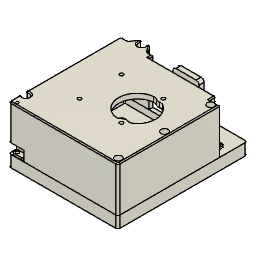
Rover Print (Autodesk Fusion 360 design; units mm, degrees)
Autodesk Fusion 360 part; units mm, degrees
sketch "Sketch1" plane through (0, 0, 0) normal (0, 1, 0) x (1, 0, 0)
  circle A0 centre (-11.34, -55.5844) radius 2
  circle A1 centre (48.2127, -47.8014) radius 2
  circle A2 centre (22.7534, 34.9922) radius 2
  circle A3 centre (-33.3857, 4.4929) radius 2
  line L0 (-55, 25) -> (10, 25)
  line L1 (10, 25) -> (18.6466, 42.3538)
  line L2 (18.6466, 42.3538) -> (53.4157, 42.3538)
  line L3 (53.4157, 42.3538) -> (53.4157, -86.2434)
  line L4 (53.4157, -86.2434) -> (-55, -86.2434)
  line L5 (-55, -86.2434) -> (-55, 25)
  circle A4 centre (48.2127, -47.8014) radius 3.5
  circle A5 centre (-11.34, -55.5844) radius 3.5
  circle A6 centre (-33.3857, 4.4929) radius 3.5
  circle A7 centre (22.7534, 34.9922) radius 3.5
  line L6 (-48, 25) -> (-43, 32)
  line L7 (-43, 32) -> (-33, 32)
  line L8 (-33, 32) -> (-28, 25)
  dimension "d1" = 4
  dimension "d2" = 4
  dimension "d3" = 4
  dimension "d4" = 4
  dimension "d8" = 7
  dimension "d9" = 7
  dimension "d10" = 7
  dimension "d11" = 7
  dimension "d61" = 7
  dimension "d62" = 5
  dimension "d63" = 5
  dimension "d64" = 20
  constraint horizontal L0
  constraint parallel L0 L2
  constraint perpendicular L2 L3
  constraint perpendicular L3 L4
  constraint perpendicular L0 L5
  constraint concentric A1 A4
  constraint concentric A0 A5
  constraint concentric A3 A6
  constraint concentric A2 A7
  constraint coincident L0 L6.start
  constraint parallel L0 L7
  constraint coincident L0 L8.end
  measures "d1" diameter of A0
  measures "d2" diameter of A1
  measures "d3" diameter of A2
  measures "d4" diameter of A3
  measures "d8" diameter of A4
  measures "d9" diameter of A5
  measures "d10" diameter of A6
  measures "d11" diameter of A7
  measures "d61" distance of L0.start L6.start
  measures "d62" horizontal distance of L6.start L6.end
  measures "d63" horizontal distance of L7.end L8.end
  measures "d64" distance of L6.start L8.end
extrude "Extrude2" add sketch "Sketch1" along normal blind 5 contours L0 L1 L2 L3 L4 L5 | L0 L6 L7 L8 | A4 | A5 | A6 | A7 makes body 1
extrude "Extrude3" add sketch "Sketch1" along normal blind 2 contours A4 | A5 | A6 | A7 bodies 1
sketch "Sketch2" plane through (0, 5, 0) normal (0, 1, 0) x (-1, 0, 0)
  circle A0 centre (-22.7534, -34.9922) radius 2
  circle A1 centre (33.3857, -4.4929) radius 2
  circle A2 centre (11.34, 55.5844) radius 2
  circle A3 centre (-48.2127, 47.8014) radius 2
  line L0 (55, 86.2434) -> (-53.4157, 86.2434)
  line L1 (-53.4157, 86.2434) -> (-53.4157, -42.3538)
  line L2 (-53.4157, -42.3538) -> (-18.6466, -42.3538)
  line L3 (-18.6466, -42.3538) -> (-10, -25)
  line L4 (48, -25) -> (55, -25)
  line L5 (55, -25) -> (55, 86.2434)
  line L6 (47, -21.0566) -> (-43.6, -21.0566)
  line L7 (-43.6, -21.0566) -> (-43.6, 82.2434)
  line L8 (-43.6, 82.2434) -> (47, 82.2434)
  line L9 (47, 82.2434) -> (47, -21.0566)
  line L10 (55, 86.2434) -> (55, -25)
  circle A4 centre (46, -20.0566) radius 1
  circle A5 centre (-42.6, -20.0566) radius 1
  circle A6 centre (-42.6, 81.2434) radius 1
  circle A7 centre (46, 81.2434) radius 1
  line L11 (33, -32) -> (43, -32)
  line L12 (43, -32) -> (48, -25)
  line L13 (-10, -25) -> (28, -25)
  line L14 (28, -25) -> (33, -32)
  line L15 (38, -32) -> (38, -29) construction
  circle A8 centre (38, -29) radius 1.3
  line L16 (-43.6, -21.0566) -> (-43.6, -11.0566) construction
  line L17 (-43.6, -11.0566) -> (-48.6, -11.0566) construction
  circle A9 centre (-48.6, -11.0566) radius 1.3
  line L18 (-48.6, -11.0566) -> (-48.6, 11.9434) construction
  circle A10 centre (-48.6, 11.9434) radius 1.3
  line L19 (-48.6, 11.9434) -> (-48.6, 34.9434) construction
  circle A11 centre (-48.6, 34.9434) radius 1.3
  line L20 (-48.6, 34.9434) -> (-48.6, 57.9434) construction
  circle A12 centre (-48.6, 57.9434) radius 1.3
  line L21 (-48.6, 57.9434) -> (-48.6, 80.9434) construction
  circle A13 centre (-48.6, 80.9434) radius 1.3
  line L22 (47, 82.2434) -> (52, 82.2434) construction
  line L23 (52, 82.2434) -> (52, 72.2434) construction
  circle A14 centre (52, 72.2434) radius 1.3
  dimension "d16" = 90.6
  dimension "d17" = 103.3
  dimension "d18" = 8
  dimension "d19" = 4
  dimension "d20" = 2
  dimension "d65" = 3
  dimension "d66" = 2.6
  dimension "d70" = 10
  dimension "d71" = 5
  dimension "d72" = 2.6
  dimension "d73" = 23
  dimension "d74" = 2.6
  dimension "d75" = 23
  dimension "d76" = 2.6
  dimension "d77" = 23
  dimension "d78" = 2.6
  dimension "d79" = 23
  dimension "d80" = 2.6
  dimension "d81" = 5
  dimension "d82" = 10
  dimension "d83" = 2.6
  constraint horizontal L6
  constraint vertical L7
  constraint horizontal L8
  constraint vertical L9
  constraint tangent L9 A4
  constraint tangent L6 A4
  constraint equal A4 A7
  constraint equal A6 A7
  constraint equal A5 A6
  constraint tangent L6 A5
  constraint tangent L7 A5
  constraint tangent L7 A6
  constraint tangent L8 A6
  constraint tangent L9 A7
  constraint tangent L8 A7
  constraint midpoint L11 L15.start
  constraint perpendicular L11 L15
  constraint coincident L15.end A8.centre
  constraint perpendicular L6 L16
  constraint perpendicular L16 L17
  constraint coincident L17.end A9.centre
  constraint perpendicular L17 L18
  constraint coincident L18.end A10.centre
  constraint parallel L18 L19
  constraint coincident L19.end A11.centre
  constraint parallel L19 L20
  constraint coincident L20.end A12.centre
  constraint parallel L20 L21
  constraint coincident L21.end A13.centre
  constraint perpendicular L9 L22
  constraint perpendicular L22 L23
  constraint coincident L23.end A14.centre
  measures "d16" distance of L6.start L6.end
  measures "d17" distance of L6.start L8.end
  measures "d18" distance of L9 L10
  measures "d19" distance of L0 L8
  measures "d20" diameter of A4
  measures "d65" distance of L15.start L15.end
  measures "d66" diameter of A8
  measures "d70" distance of L6.end L16.end
  measures "d71" distance of L16.end L17.end
  measures "d72" diameter of A9
  measures "d73" distance of L17.end L18.end
  measures "d74" diameter of A10
  measures "d75" distance of L18.end L19.end
  measures "d76" diameter of A11
  measures "d77" distance of L19.end L20.end
  measures "d78" diameter of A12
  measures "d79" distance of L20.end L21.end
  measures "d80" diameter of A13
  measures "d81" distance of L8.end L22.end
  measures "d82" distance of L22.end L23.end
  measures "d83" diameter of A14
extrude "Extrude4" add sketch "Sketch2" along normal blind 6.5 contours L0 L1 L2 L3 L4 L5 L10 L11 L12 L13 L14 | L6 L9 A4 | L6 L7 A5 | L8 L9 A7 | L7 L8 A6 | A8 | A9 | A10 | A11 | A12 | A13 | A14 bodies 1
extrude "Extrude5" cut sketch "Sketch1" against normal blind 9.5 from surface at 11.5 contours A4 | A7 bodies 1
extrude "Extrude6" cut sketch "Sketch1" against normal blind 3 from surface at 5 contours A5 | A6 bodies 1
fillet "Fillet1" radius 2 7 edges at (-55, 8.25, -25) (-55, 2.5, -25) (-55, 5.75, 86.2434) (53.4157, 5.75, 86.2434) (53.4157, 5.75, -42.3538) (18.6466, 5.75, -42.3538) (10, 2.5, -25) on bodies 1
sketch "Sketch3" plane through (0, 11.5, 0) normal (0, 1, 0) x (-1, 0, 0)
  arc A0 (-19.8846, -42.3538) -> (-18.0945, -41.2457) centre (-19.8846, -40.3538) ccw
  line L0 (-18.0945, -41.2457) -> (-10.5521, -26.1081)
  line L1 (48, -25) -> (53, -25)
  arc A1 (53, -25) -> (55, -23) centre (53, -23) ccw
  line L2 (55, -23) -> (55, 84.2434)
  arc A2 (55, 84.2434) -> (53, 86.2434) centre (53, 84.2434) ccw
  line L3 (53, 86.2434) -> (-51.4157, 86.2434)
  arc A3 (-51.4157, 86.2434) -> (-53.4157, 84.2434) centre (-51.4157, 84.2434) ccw
  line L4 (-53.4157, 84.2434) -> (-53.4157, -40.3538)
  arc A4 (-53.4157, -40.3538) -> (-51.4157, -42.3538) centre (-51.4157, -40.3538) ccw
  line L5 (-51.4157, -42.3538) -> (-19.8846, -42.3538)
  arc A5 (46, -21.0566) -> (47, -20.0566) centre (46, -20.0566) ccw
  line L6 (46, -21.0566) -> (-42.6, -21.0566)
  arc A6 (-43.6, -20.0566) -> (-42.6, -21.0566) centre (-42.6, -20.0566) ccw
  line L7 (-43.6, -20.0566) -> (-43.6, 81.2434)
  arc A7 (-42.6, 82.2434) -> (-43.6, 81.2434) centre (-42.6, 81.2434) ccw
  line L8 (-42.6, 82.2434) -> (46, 82.2434)
  arc A8 (47, 81.2434) -> (46, 82.2434) centre (46, 81.2434) ccw
  line L9 (47, 81.2434) -> (47, -20.0566)
  circle A9 centre (-22.7534, -34.9922) radius 3.5
  circle A10 centre (-48.2127, 47.8014) radius 3.5
  line L10 (46, 82.2434) -> (46, 80.7434) construction
  line L11 (46, 80.7434) -> (42, 80.7434) construction
  line L12 (42, 80.7434) -> (52, 80.7434)
  line L13 (52, 80.7434) -> (52, 85.7434)
  line L14 (52, 85.7434) -> (42, 85.7434)
  line L15 (42, 85.7434) -> (42, 80.7434)
  circle A11 centre (49.5, 83.2434) radius 1.6
  circle A12 centre (49.5, 83.2434) radius 1.3
  line L16 (-43.6, -20.0566) -> (-41.6, -20.0566) construction
  line L17 (-41.6, -20.0566) -> (-41.6, -16.0566) construction
  line L18 (-41.6, -16.0566) -> (-46.6, -16.0566)
  line L19 (-46.6, -16.0566) -> (-46.6, -26.0566)
  line L20 (-46.6, -26.0566) -> (-41.6, -26.0566)
  line L21 (-41.6, -26.0566) -> (-41.6, -16.0566)
  circle A13 centre (-44.1, -23.5566) radius 1.6
  circle A14 centre (-44.1, -23.5566) radius 1.3
  arc A15 (-8.762, -25) -> (-10.5521, -26.1081) centre (-8.762, -27) ccw
  line L22 (-8.762, -25) -> (28, -25)
  line L23 (28, -25) -> (33, -32)
  line L24 (33, -32) -> (43, -32)
  line L25 (43, -32) -> (48, -25)
  dimension "d31" = 1.5
  dimension "d32" = 10
  dimension "d33" = 5
  dimension "d34" = 3.2
  dimension "d35" = 2.6
  dimension "d42" = 2
  dimension "d43" = 4
  dimension "d44" = 5
  dimension "d45" = 10
  dimension "d46" = 3.2
  dimension "d47" = 2.6
  dimension "d48" = 2.5
  dimension "d49" = 2.5
  dimension "d50" = 2.5
  dimension "d51" = 2.5
  constraint coincident L8.end A8.end
  constraint perpendicular L8 L10
  constraint perpendicular L10 L11
  constraint horizontal L12
  constraint vertical L13
  constraint horizontal L14
  constraint vertical L15
  constraint concentric A11 A12
  constraint coincident A6.start L7.start
  constraint perpendicular L7 L16
  constraint perpendicular L16 L17
  constraint horizontal L18
  constraint vertical L19
  constraint horizontal L20
  constraint vertical L21
  constraint concentric A13 A14
  measures "d31" distance of L8.end L10.end
  measures "d32" distance of L11.end L12.end
  measures "d33" distance of L11.end L14.end
  measures "d34" diameter of A11
  measures "d35" diameter of A12
  measures "d42" distance of A6.start L16.end
  measures "d43" distance of L16.end L17.end
  measures "d44" distance of L17.end L18.end
  measures "d45" distance of L17.end L20.end
  measures "d46" diameter of A13
  measures "d47" diameter of A14
  measures "d48" distance of L13 A11.centre
  measures "d49" distance of L14 A11.centre
  measures "d50" distance of L20 A13.centre
  measures "d51" distance of L19 A13.centre
extrude "Extrude7" cut sketch "Sketch3" against normal blind 7 contours A12 bodies 1
extrude "Extrude8" add sketch "Sketch3" along normal blind 2 separate body contours L8 A8 L9 L12 L15 | L8 A8 L9 L12 L13 L14 L15 makes body 2
fillet "Fillet2" radius 1 4 edges at (-42, 12.5, 85.7434) (-52, 12.5, 85.7434) (-52, 12.5, 80.7434) (-42, 12.5, 80.7434) on bodies 2
extrude "Extrude9" cut sketch "Sketch3" against normal blind 7 contours A14 bodies 1
extrude "Extrude10" add sketch "Sketch3" along normal blind 2 separate body contours L6 A6 L7 L18 L19 L20 L21 | L6 A6 L7 L18 L21 makes body 3
fillet "Fillet3" radius 1 4 edges at (46.6, 12.5, -16.0566) (41.6, 12.5, -16.0566) (41.6, 12.5, -26.0566) (46.6, 12.5, -26.0566) on bodies 3
fillet "Fillet4" radius 2 6 edges at (-48, 2.5, -25) (-48, 8.25, -25) (-43, 5.75, -32) (-33, 5.75, -32) (-28, 2.5, -25) (-28, 8.25, -25) on bodies 1
extrude "Extrude11" cut sketch "Sketch2" against normal blind 7 from surface at 6.5 contours A8 bodies 1
extrude "Extrude12" cut sketch "Sketch2" against normal blind 7 from surface at 6.5 contours A9 | A10 | A11 | A12 | A13 | A14 bodies 1
sketch "Sketch4" plane through (0, 11.5, 0) normal (0, 1, 0) x (-1, 0, 0)
  circle A0 centre (-48.6, 34.9434) radius 1.3
  circle A1 centre (52, 72.2434) radius 1.3
  circle A2 centre (-48.6, 11.9434) radius 1.3
  circle A3 centre (-48.6, 57.9434) radius 1.3
  circle A4 centre (-48.6, 80.9434) radius 1.3
  circle A5 centre (-48.6, -11.0566) radius 1.3
  circle A6 centre (38, -29) radius 1.3
  circle A7 centre (-44.1, -23.5566) radius 1.3
  circle A8 centre (49.5, 83.2434) radius 1.3
  arc A9 (32.4018, -31.1625) -> (34.0292, -32) centre (34.0292, -30) ccw
  line L0 (34.0292, -32) -> (41.9708, -32)
  arc A10 (41.9708, -32) -> (43.5982, -31.1625) centre (41.9708, -30) ccw
  line L1 (43.5982, -31.1625) -> (47.4018, -25.8375)
  arc A11 (49.0292, -25) -> (47.4018, -25.8375) centre (49.0292, -27) ccw
  line L2 (49.0292, -25) -> (53, -25)
  arc A12 (53, -25) -> (55, -23) centre (53, -23) ccw
  line L3 (55, -23) -> (55, 84.2434)
  arc A13 (55, 84.2434) -> (53, 86.2434) centre (53, 84.2434) ccw
  line L4 (53, 86.2434) -> (-51.4157, 86.2434)
  arc A14 (-51.4157, 86.2434) -> (-53.4157, 84.2434) centre (-51.4157, 84.2434) ccw
  line L5 (-53.4157, 84.2434) -> (-53.4157, -40.3538)
  arc A15 (-53.4157, -40.3538) -> (-51.4157, -42.3538) centre (-51.4157, -40.3538) ccw
  line L6 (-51.4157, -42.3538) -> (-19.8846, -42.3538)
  arc A16 (-19.8846, -42.3538) -> (-18.0945, -41.2457) centre (-19.8846, -40.3538) ccw
  line L7 (-18.0945, -41.2457) -> (-10.5521, -26.1081)
  arc A17 (-8.762, -25) -> (-10.5521, -26.1081) centre (-8.762, -27) ccw
  line L8 (-8.762, -25) -> (26.9708, -25)
  arc A18 (28.5982, -25.8375) -> (26.9708, -25) centre (26.9708, -27) ccw
  line L9 (28.5982, -25.8375) -> (32.4018, -31.1625)
  arc A19 (46, -21.0566) -> (47, -20.0566) centre (46, -20.0566) ccw
  line L10 (46, -21.0566) -> (-42.6, -21.0566)
  arc A20 (-43.6, -20.0566) -> (-42.6, -21.0566) centre (-42.6, -20.0566) ccw
  line L11 (-43.6, -20.0566) -> (-43.6, 81.2434)
  arc A21 (-42.6, 82.2434) -> (-43.6, 81.2434) centre (-42.6, 81.2434) ccw
  line L12 (-42.6, 82.2434) -> (46, 82.2434)
  arc A22 (47, 81.2434) -> (46, 82.2434) centre (46, 81.2434) ccw
  line L13 (47, 81.2434) -> (47, -20.0566)
  circle A23 centre (-22.7534, -34.9922) radius 3.5
  circle A24 centre (-48.2127, 47.8014) radius 3.5
  line L14 (47, -20.0566) -> (55, -20.0566)
  line L15 (23, -21.0566) -> (23, -25)
  line L16 (-43.6, -15.0178) -> (-53.4157, -15.0178)
  line L17 (47, 59.5753) -> (55, 59.5753)
  circle A25 centre (52, 72.2434) radius 3.5
  circle A26 centre (38, -29) radius 3.5
  circle A27 centre (-48.6, -11.0566) radius 3.5
  circle A28 centre (-48.6, 34.9434) radius 3.5
  circle A29 centre (-48.6, 80.9434) radius 3.5
  dimension "d117" = 7
  dimension "d118" = 7
  dimension "d119" = 7
  dimension "d120" = 7
  dimension "d121" = 7
  dimension "d133" = 24
  constraint coincident A19.end L13.end
  constraint coincident L3 L14.end
  constraint perpendicular L3 L14
  constraint coincident L10 L15.start
  constraint coincident L8 L15.end
  constraint perpendicular L8 L15
  constraint coincident L11 L16.start
  constraint coincident L5 L16.end
  constraint perpendicular L5 L16
  constraint coincident L13 L17.start
  constraint coincident L3 L17.end
  constraint perpendicular L3 L17
  constraint concentric A1 A25
  constraint concentric A6 A26
  constraint concentric A5 A27
  constraint concentric A0 A28
  constraint concentric A4 A29
  measures "d117" diameter of A25
  measures "d118" diameter of A26
  measures "d119" diameter of A27
  measures "d120" diameter of A28
  measures "d121" diameter of A29
  measures "d133" horizontal distance of A19.end L15.start
extrude "Extrude13" add sketch "Sketch4" along normal blind 40 separate body contours A2 | A3 | A9 L0 A10 L1 A11 L2 A12 L3 L8 A18 L9 A19 L10 L14 L15 A26 | L0 A26 | L3 A13 L4 A14 L5 L11 A21 L12 A22 L13 L16 L17 A25 | L3 A25 | A24 | A27 | A28 | A29 picked at (37.9676, -31.4321) picked at (54.4333, 72.2434) makes body 4 at (-38.3333, 24.8333, -21.0566) makes body 5 at (-18.1948, 24.8333, 86.2434)
extrude "Extrude14" add sketch "Sketch4" along normal blind 5 from surface at 40 contours A2 | A3 | A9 L0 A10 L1 A11 L2 A12 L3 L8 A18 L9 A19 L10 L14 L15 A26 | L0 A26 | A19 L10 A20 L11 A21 L12 A22 L13 | L3 L13 L14 L17 | L3 A13 L4 A14 L5 L11 A21 L12 A22 L13 L16 L17 A25 | L3 A25 | A24 | A27 | A28 | A29 picked at (37.9676, -31.4321) picked at (54.4333, 72.2434) bodies 4 5
sketch "Sketch5" plane through (0, 51.5, 0) normal (0, -1, 0) x (1, 0, 0)
  line L0 (-55, -20.0566) -> (-47, -20.0566)
  arc A0 (-47, -20.0566) -> (-46, -21.0566) centre (-46, -20.0566) ccw
  line L1 (-46, -21.0566) -> (-23, -21.0566)
  line L2 (-23, -21.0566) -> (42.6, -21.0566)
  arc A1 (42.6, -21.0566) -> (43.6, -20.0566) centre (42.6, -20.0566) ccw
  line L3 (43.6, -20.0566) -> (43.6, -15.0178)
  line L4 (43.6, -15.0178) -> (43.6, 81.2434)
  arc A2 (43.6, 81.2434) -> (42.6, 82.2434) centre (42.6, 81.2434) ccw
  line L5 (42.6, 82.2434) -> (-46, 82.2434)
  arc A3 (-46, 82.2434) -> (-47, 81.2434) centre (-46, 81.2434) ccw
  line L6 (-47, 81.2434) -> (-47, 59.5753)
  line L7 (-47, 59.5753) -> (-55, 59.5753)
  line L8 (-55, 59.5753) -> (-55, -20.0566)
  line L9 (-1.1187, -54.3751) -> (-1.1187, 110.6249) construction
  circle A4 centre (-1.1187, 28.1249) radius 29.5 construction
  line L10 (-1.1187, 28.1249) -> (19.7409, 7.2652) construction
  line L11 (-1.1187, 28.1249) -> (20, 28.1249) construction
  circle A5 centre (19.7409, 7.2652) radius 1.75
  circle A6 centre (19.7409, 48.9845) radius 1.75
  circle A7 centre (-21.9784, 48.9845) radius 1.75
  circle A8 centre (-21.9784, 7.2652) radius 1.75
  dimension "d92" = 59
  dimension "d93" = 45
  dimension "d94" = 3.5
  dimension "d96" = 360
  constraint perpendicular L5 L9
  constraint midpoint L9 A4.centre
  constraint horizontal L11
  constraint coincident A4.centre L10.start
  constraint coincident A4 L10.end
  constraint coincident L10.end A5.centre
  measures "d92" diameter of A4
  measures "d93" angle of L10 L11
  measures "d94" diameter of A5
extrude "Extrude15" cut sketch "Sketch5" along normal blind 20 from surface at -5 contours A5 | A6 | A7 | A8 bodies 4
sketch "Sketch6" plane through (0, 56.5, 0) normal (0, 1, 0) x (-1, 0, 0)
  circle A0 centre (21.9784, 7.2652) radius 1.75
  circle A1 centre (21.9784, 48.9845) radius 1.75
  circle A2 centre (-19.7409, 7.2652) radius 1.75
  circle A3 centre (-19.7409, 48.9845) radius 1.75
  circle A4 centre (49.5, 83.2434) radius 1.3
  circle A5 centre (52, 72.2434) radius 1.3
  circle A6 centre (-48.6, 80.9434) radius 1.3
  circle A7 centre (-48.6, -11.0566) radius 1.3
  circle A8 centre (38, -29) radius 1.3
  circle A9 centre (-48.6, 34.9434) radius 1.3
  line L0 (-43.6, -15.0178) -> (-43.6, -20.0566)
  arc A10 (-43.6, -20.0566) -> (-42.6, -21.0566) centre (-42.6, -20.0566) ccw
  line L1 (-42.6, -21.0566) -> (23, -21.0566)
  line L2 (23, -21.0566) -> (23, -25)
  line L3 (23, -25) -> (26.9708, -25)
  arc A11 (28.5982, -25.8375) -> (26.9708, -25) centre (26.9708, -27) ccw
  line L4 (28.5982, -25.8375) -> (32.4018, -31.1625)
  arc A12 (32.4018, -31.1625) -> (34.0292, -32) centre (34.0292, -30) ccw
  line L5 (34.0292, -32) -> (41.9708, -32)
  arc A13 (41.9708, -32) -> (43.5982, -31.1625) centre (41.9708, -30) ccw
  line L6 (43.5982, -31.1625) -> (47.4018, -25.8375)
  arc A14 (49.0292, -25) -> (47.4018, -25.8375) centre (49.0292, -27) ccw
  line L7 (49.0292, -25) -> (53, -25)
  arc A15 (53, -25) -> (55, -23) centre (53, -23) ccw
  line L8 (55, -23) -> (55, 84.2434)
  arc A16 (55, 84.2434) -> (53, 86.2434) centre (53, 84.2434) ccw
  line L9 (53, 86.2434) -> (-51.4157, 86.2434)
  arc A17 (-51.4157, 86.2434) -> (-53.4157, 84.2434) centre (-51.4157, 84.2434) ccw
  line L10 (-53.4157, 84.2434) -> (-53.4157, -15.0178)
  line L11 (-53.4157, -15.0178) -> (-43.6, -15.0178)
  circle A18 centre (-48.6, -11.0566) radius 3.5
  circle A19 centre (-48.6, 11.9434) radius 3.5
  circle A20 centre (-48.6, 34.9434) radius 3.5
  circle A21 centre (-48.6, 57.9434) radius 3.5
  circle A22 centre (-48.6, 80.9434) radius 3.5
  circle A23 centre (52, 72.2434) radius 3.5
  circle A24 centre (38, -29) radius 3.5
  dimension "d100" = 7
  dimension "d101" = 7
  dimension "d102" = 7
  dimension "d103" = 7
  dimension "d104" = 7
  dimension "d105" = 7
  dimension "d108" = 7
  constraint concentric A7 A18
  constraint concentric A9 A20
  constraint concentric A6 A22
  constraint concentric A5 A23
  constraint concentric A8 A24
  measures "d100" diameter of A18
  measures "d101" diameter of A19
  measures "d102" diameter of A20
  measures "d103" diameter of A21
  measures "d104" diameter of A22
  measures "d105" diameter of A23
  measures "d108" diameter of A24
sketch "Sketch7" plane through (0, 11.5, 0) normal (0, -1, 0) x (1, 0, 0)
  circle A0 centre (-52, 72.2434) radius 1.3
  circle A1 centre (48.6, -11.0566) radius 1.3
  circle A2 centre (48.6, 80.9434) radius 1.3
  circle A3 centre (48.6, 34.9434) radius 1.3
  circle A4 centre (-49.5, 83.2434) radius 1.3
  line L0 (-47, 59.5753) -> (-47, 81.2434)
  arc A5 (-46, 82.2434) -> (-47, 81.2434) centre (-46, 81.2434) ccw
  line L1 (-46, 82.2434) -> (42.6, 82.2434)
  arc A6 (43.6, 81.2434) -> (42.6, 82.2434) centre (42.6, 81.2434) ccw
  line L2 (43.6, 81.2434) -> (43.6, -15.0178)
  line L3 (43.6, -15.0178) -> (53.4157, -15.0178)
  line L4 (53.4157, -15.0178) -> (53.4157, 84.2434)
  arc A7 (53.4157, 84.2434) -> (51.4157, 86.2434) centre (51.4157, 84.2434) ccw
  line L5 (51.4157, 86.2434) -> (-53, 86.2434)
  arc A8 (-53, 86.2434) -> (-55, 84.2434) centre (-53, 84.2434) ccw
  line L6 (-55, 84.2434) -> (-55, 59.5753)
  line L7 (-55, 59.5753) -> (-47, 59.5753)
  line L8 (-47, 79) -> (-55, 79)
  line L9 (-40.1248, 82.2434) -> (-40.1248, 86.2434)
  constraint coincident L0 L8.start
  constraint coincident L6 L8.end
  constraint perpendicular L6 L8
  constraint coincident L1 L9.start
  constraint coincident L5 L9.end
  constraint perpendicular L5 L9
extrude "Extrude16" cut sketch "Sketch7" against normal blind 10 contours A4 | L0 A5 L1 L5 A8 L6 L8 L9 bodies 4
extrude "Extrude17" cut sketch "Sketch6" against normal blind 45 contours L8 A23 | L5 A24 | A18 | A20 | A22 picked at (54.4333, 72.2434) picked at (37.9676, -31.4321) bodies 4
extrude "Extrude18" add sketch "Sketch4" along normal blind 2 contours L0 A26 | L3 A25 | A27 | A28 | A29 picked at (37.9676, -31.4321) picked at (54.4333, 72.2434) bodies 4
fillet "Fillet5" radius 1 2 edges at (-55, 34, 70.4406) (-55, 34, 74.0462) on bodies 4
fillet "Fillet6" radius 1 2 edges at (-36.1972, 34, -32) (-39.8028, 34, -32) on bodies 4
fillet "Fillet7" radius 1 26 edges at (-23, 56.5, -23.0283) (43.6, 56.5, -17.5372) (43.3071, 56.5, -20.7637) (9.8, 56.5, -21.0566) (-24.9854, 56.5, -25) (-27.8859, 56.5, -25.2217) (-30.5, 56.5, -28.5) (-33.06, 56.5, -31.7494) (-34.8011, 56.5, -31.5512) (-38, 56.5, -25.5) (-41.1989, 56.5, -31.5512) (-42.94, 56.5, -31.7494) (-45.5, 56.5, -28.5) (-48.1141, 56.5, -25.2217) (-51.0146, 56.5, -25) (-54.4142, 56.5, -24.4142) (-55, 56.5, 22.6061) (-54.527, 56.5, 69.0621) (-48.5, 56.5, 72.2434) (-54.527, 56.5, 75.4247) (-55, 56.5, 80.259) (-54.4142, 56.5, 85.6576) (-0.7922, 56.5, 86.2434) (52.8299, 56.5, 85.6576) (53.4157, 56.5, 34.6128) (48.5078, 56.5, -15.0178) on bodies 4
sketch "Sketch8" plane through (0, 56.5, 0) normal (0, 1, 0) x (-1, 0, 0)
  line L0 (-52.4157, -14.0178) -> (-50.4658, -14.0178)
  arc A0 (-46.7342, -14.0178) -> (-50.4658, -14.0178) centre (-48.6, -11.0566) ccw
  line L1 (-46.7342, -14.0178) -> (-42.6, -14.0178)
  line L2 (-42.6, -14.0178) -> (-42.6, -20.0566)
  line L3 (-42.6, -20.0566) -> (24, -20.0566)
  line L4 (24, -20.0566) -> (24, -24)
  line L5 (24, -24) -> (26.9708, -24)
  arc A1 (29.412, -25.2563) -> (26.9708, -24) centre (26.9708, -27) ccw
  line L6 (29.412, -25.2563) -> (33.2155, -30.5812)
  arc A2 (33.2155, -30.5812) -> (33.9679, -30.9981) centre (34.0292, -30) ccw
  arc A3 (42.0321, -30.9981) -> (33.9679, -30.9981) centre (38, -29) ccw
  arc A4 (42.0321, -30.9981) -> (42.7845, -30.5812) centre (41.9708, -30) ccw
  line L7 (42.7845, -30.5812) -> (46.588, -25.2563)
  arc A5 (49.0292, -24) -> (46.588, -25.2563) centre (49.0292, -27) ccw
  line L8 (49.0292, -24) -> (53, -24)
  arc A6 (53, -24) -> (54, -23) centre (53, -23) ccw
  line L9 (54, -23) -> (54, 68.2123)
  arc A7 (54, 76.2746) -> (54, 68.2123) centre (52, 72.2434) ccw
  line L10 (54, 76.2746) -> (54, 84.2434)
  arc A8 (54, 84.2434) -> (53, 85.2434) centre (53, 84.2434) ccw
  line L11 (53, 85.2434) -> (-51.4157, 85.2434)
  arc A9 (-51.4157, 85.2434) -> (-52.4157, 84.2434) centre (-51.4157, 84.2434) ccw
  line L12 (-52.4157, 84.2434) -> (-52.4157, -14.0178)
  circle A10 centre (-48.6, 34.9434) radius 3.5
  circle A11 centre (-48.6, 80.9434) radius 3.5
  circle A12 centre (21.9784, 7.2652) radius 1.75
  circle A13 centre (21.9784, 48.9845) radius 1.75
  circle A14 centre (-19.7409, 7.2652) radius 1.75
  circle A15 centre (-19.7409, 48.9845) radius 1.75
  circle A16 centre (49.5, 83.2434) radius 1.3
  line L13 (-43.6, 82.2) -> (-33.6, 82.2) construction
  line L14 (-33.6, 82.2) -> (-33.6, 47.2) construction
  line L15 (-33.6, 47.2) -> (3.4, 47.2) construction
  line L16 (3.4, 47.2) -> (3.4, 10.2) construction
  line L17 (3.4, 10.2) -> (-33.6, 10.2) construction
  line L18 (-33.6, 10.2) -> (-33.6, 47.2) construction
  circle A17 centre (-15.1, 28.7) radius 18.5
  circle A18 centre (-19.7409, 48.9845) radius 5
  circle A19 centre (-19.7409, 7.2652) radius 5
  dimension "d124" = 10
  dimension "d125" = 35
  dimension "d126" = 37
  dimension "d127" = 37
  dimension "d128" = 37
  dimension "d173" = 10
  dimension "d174" = 10
  constraint parallel L11 L13
  constraint perpendicular L13 L14
  constraint horizontal L15
  constraint vertical L16
  constraint horizontal L17
  constraint vertical L18
  constraint concentric A15 A18
  constraint concentric A14 A19
  measures "d124" distance of L13.start L13.end
  measures "d125" distance of L13.end L14.end
  measures "d126" distance of L14.end L15.end
  measures "d127" distance of L14.end L17.end
  measures "d128" diameter of A17
  measures "d173" diameter of A18
  measures "d174" diameter of A19
extrude "Extrude19" cut sketch "Sketch8" against normal blind 10 contours A17 A18 A19 bodies 4
fillet "Fillet8" radius 5 3 edges at (23.171, 54, 45.3466) (23.171, 54, 45.3466) (15.0703, 54, 47.2) on bodies 4
sketch "Sketch9" plane through (0, 11.5, 0) normal (0, 1, 0) x (-1, 0, 0)
  circle A0 centre (-48.6, 34.9434) radius 1.3
  circle A1 centre (52, 72.2434) radius 1.3
  circle A2 centre (-48.6, 11.9434) radius 1.3
  circle A3 centre (-48.6, 57.9434) radius 1.3
  circle A4 centre (-48.6, 80.9434) radius 1.3
  circle A5 centre (-48.6, -11.0566) radius 1.3
  circle A6 centre (38, -29) radius 1.3
  circle A7 centre (-44.1, -23.5566) radius 1.3
  circle A8 centre (49.5, 83.2434) radius 1.3
  arc A9 (32.4018, -31.1625) -> (34.0292, -32) centre (34.0292, -30) ccw
  line L0 (34.0292, -32) -> (41.9708, -32)
  arc A10 (41.9708, -32) -> (43.5982, -31.1625) centre (41.9708, -30) ccw
  line L1 (43.5982, -31.1625) -> (47.4018, -25.8375)
  arc A11 (49.0292, -25) -> (47.4018, -25.8375) centre (49.0292, -27) ccw
  line L2 (49.0292, -25) -> (53, -25)
  arc A12 (53, -25) -> (55, -23) centre (53, -23) ccw
  line L3 (55, -23) -> (55, 84.2434)
  arc A13 (55, 84.2434) -> (53, 86.2434) centre (53, 84.2434) ccw
  line L4 (53, 86.2434) -> (-51.4157, 86.2434)
  arc A14 (-51.4157, 86.2434) -> (-53.4157, 84.2434) centre (-51.4157, 84.2434) ccw
  line L5 (-53.4157, 84.2434) -> (-53.4157, -40.3538)
  arc A15 (-53.4157, -40.3538) -> (-51.4157, -42.3538) centre (-51.4157, -40.3538) ccw
  line L6 (-51.4157, -42.3538) -> (-19.8846, -42.3538)
  arc A16 (-19.8846, -42.3538) -> (-18.0945, -41.2457) centre (-19.8846, -40.3538) ccw
  line L7 (-18.0945, -41.2457) -> (-10.5521, -26.1081)
  arc A17 (-8.762, -25) -> (-10.5521, -26.1081) centre (-8.762, -27) ccw
  line L8 (-8.762, -25) -> (26.9708, -25)
  arc A18 (28.5982, -25.8375) -> (26.9708, -25) centre (26.9708, -27) ccw
  line L9 (28.5982, -25.8375) -> (32.4018, -31.1625)
  arc A19 (46, -21.0566) -> (47, -20.0566) centre (46, -20.0566) ccw
  line L10 (46, -21.0566) -> (-42.6, -21.0566)
  arc A20 (-43.6, -20.0566) -> (-42.6, -21.0566) centre (-42.6, -20.0566) ccw
  line L11 (-43.6, -20.0566) -> (-43.6, 81.2434)
  arc A21 (-42.6, 82.2434) -> (-43.6, 81.2434) centre (-42.6, 81.2434) ccw
  line L12 (-42.6, 82.2434) -> (46, 82.2434)
  arc A22 (47, 81.2434) -> (46, 82.2434) centre (46, 81.2434) ccw
  line L13 (47, 81.2434) -> (47, -20.0566)
  circle A23 centre (-22.7534, -34.9922) radius 3.5
  circle A24 centre (-48.2127, 47.8014) radius 3.5
  line L14 (0, 0) -> (0, -36) construction
  constraint coincident L14.start origin
  constraint vertical L14
sketch "Sketch10" plane through (0, 0, -25) normal (0, 0, -1) x (-1, 0, 0)
  line L0 (26.9708, 5) -> (26.9708, 11.5)
  line L1 (26.9708, 11.5) -> (-8.762, 11.5)
  line L2 (-8.762, 11.5) -> (-8.762, 5)
  line L3 (-8.762, 5) -> (26.9708, 5)
  circle A0 centre (-4, 8) radius 1.3
  line L4 (-4, 8) -> (16, 8) construction
  circle A1 centre (16, 8) radius 1.3
  line L5 (6, 8) -> (6, 3) construction
  circle A2 centre (6, 3) radius 1.3
  line L6 (6, 0) -> (0, 0)
  line L7 (0, 0) -> (-7, 5)
  line L8 (12, 0) -> (19, 5)
  line L9 (6, 0) -> (12, 0)
  line L10 (-7, 5) -> (-7, 11.5)
  line L11 (19, 5) -> (19, 11.5)
  dimension "d134" = 2.6
  dimension "d135" = 20
  dimension "d136" = 2.6
  dimension "d137" = 5
  dimension "d138" = 2.6
  constraint coincident A0.centre L4.start
  constraint horizontal L4
  constraint coincident L4.end A1.centre
  constraint midpoint L4 L5.start
  constraint perpendicular L4 L5
  constraint coincident L5.end A2.centre
  constraint coincident L6.end L7.start
  constraint horizontal L6
  constraint coincident L3 L7.end
  constraint symmetric L5 L6.start L9.start
  constraint symmetric L5 L6.end L8.start
  constraint symmetric L5 L7.end L8.end
  constraint coincident L1 L10.end
  constraint perpendicular L1 L10
  constraint coincident L1 L11.end
  constraint perpendicular L1 L11
  measures "d134" diameter of A0
  measures "d135" distance of A0.centre L4.end
  measures "d136" diameter of A1
  measures "d137" distance of L5.start L5.end
  measures "d138" diameter of A2
extrude "Extrude20" add sketch "Sketch10" along normal blind 15 separate body contours L3 L6 L7 L8 L9 | L1 L3 L10 L11 | A0 | A1 | A2 makes body 6
move_body "Move1" bodies 6 to x (1, 0, 0) y (0, 1, 0) z (0, 0, 1) at (6, 0, 0)
combine "Combine1" operation add target body 1 tool bodies 6
sketch "Sketch11" plane through (0, 11.5, 0) normal (0, 1, 0) x (-1, 0, 0)
  circle A0 centre (-48.2127, 47.8014) radius 3.5
  circle A1 centre (-22.7534, -34.9922) radius 3.5
  arc A2 (46, -21.0566) -> (47, -20.0566) centre (46, -20.0566) ccw
  line L0 (46, -21.0566) -> (-42.6, -21.0566)
  arc A3 (-43.6, -20.0566) -> (-42.6, -21.0566) centre (-42.6, -20.0566) ccw
  line L1 (-43.6, -20.0566) -> (-43.6, 81.2434)
  arc A4 (-42.6, 82.2434) -> (-43.6, 81.2434) centre (-42.6, 81.2434) ccw
  line L2 (-42.6, 82.2434) -> (46, 82.2434)
  arc A5 (47, 81.2434) -> (46, 82.2434) centre (46, 81.2434) ccw
  line L3 (47, 81.2434) -> (47, -20.0566)
  line L4 (-13, -31.021) -> (-13, -40)
  line L5 (-13, -40) -> (13, -40)
  line L6 (13, -40) -> (13, -25)
  line L7 (13, -25) -> (26.9708, -25)
  arc A6 (28.5982, -25.8375) -> (26.9708, -25) centre (26.9708, -27) ccw
  line L8 (28.5982, -25.8375) -> (32.4018, -31.1625)
  arc A7 (32.4018, -31.1625) -> (34.0292, -32) centre (34.0292, -30) ccw
  line L9 (34.0292, -32) -> (41.9708, -32)
  arc A8 (41.9708, -32) -> (43.5982, -31.1625) centre (41.9708, -30) ccw
  line L10 (43.5982, -31.1625) -> (47.4018, -25.8375)
  arc A9 (49.0292, -25) -> (47.4018, -25.8375) centre (49.0292, -27) ccw
  line L11 (49.0292, -25) -> (53, -25)
  arc A10 (53, -25) -> (55, -23) centre (53, -23) ccw
  line L12 (55, -23) -> (55, 84.2434)
  arc A11 (55, 84.2434) -> (53, 86.2434) centre (53, 84.2434) ccw
  line L13 (53, 86.2434) -> (-51.4157, 86.2434)
  arc A12 (-51.4157, 86.2434) -> (-53.4157, 84.2434) centre (-51.4157, 84.2434) ccw
  line L14 (-53.4157, 84.2434) -> (-53.4157, -40.3538)
  arc A13 (-53.4157, -40.3538) -> (-51.4157, -42.3538) centre (-51.4157, -40.3538) ccw
  line L15 (-51.4157, -42.3538) -> (-19.8846, -42.3538)
  arc A14 (-19.8846, -42.3538) -> (-18.0945, -41.2457) centre (-19.8846, -40.3538) ccw
  line L16 (-18.0945, -41.2457) -> (-13, -31.021)
  circle A15 centre (49.5, 83.2434) radius 1.3
  circle A16 centre (-44.1, -23.5566) radius 1.3
  circle A17 centre (38, -29) radius 1.3
  circle A18 centre (-48.6, -11.0566) radius 1.3
  circle A19 centre (-48.6, 80.9434) radius 1.3
  circle A20 centre (-48.6, 57.9434) radius 1.3
  circle A21 centre (-48.6, 11.9434) radius 1.3
  circle A22 centre (52, 72.2434) radius 1.3
  circle A23 centre (-48.6, 34.9434) radius 1.3
  circle A24 centre (0, -31) radius 1.3
  line L17 (13, -40) -> (13, -35) construction
  line L18 (13, -35) -> (-13, -35)
  line L19 (0, -35) -> (0, -31) construction
  line L20 (0, -31) -> (-9, -31) construction
  circle A25 centre (-9, -31) radius 1.3
  line L21 (0, -31) -> (9, -31) construction
  circle A26 centre (9, -31) radius 1.3
  line L22 (-13, -35) -> (-13, -25)
  line L23 (-13, -25) -> (13, -25)
  dimension "d141" = 2.6
  dimension "d142" = 5
  dimension "d143" = 4
  dimension "d144" = 2.6
  dimension "d145" = 9
  dimension "d146" = 2.6
  dimension "d147" = 10
  constraint coincident L5.end L6.start
  constraint perpendicular L5 L17
  constraint coincident L4 L18.end
  constraint perpendicular L4 L18
  constraint midpoint L18 L19.start
  constraint perpendicular L18 L19
  constraint coincident A24.centre L19.end
  constraint perpendicular L19 L20
  constraint coincident L20.end A25.centre
  constraint perpendicular L19 L21
  constraint coincident L21.end A26.centre
  constraint perpendicular L18 L22
  constraint coincident L6.end L7.start
  measures "d141" diameter of A24
  measures "d142" distance of L5.end L17.end
  measures "d143" distance of L19.start A24.centre
  measures "d144" diameter of A25
  measures "d145" distance of A24.centre L21.end
  measures "d146" diameter of A26
  measures "d147" distance of L18.end L22.end
extrude "Extrude21" add sketch "Sketch11" along normal blind 5 contours L4 L6 L18 L22 L23 | L4 L5 L6 L18 bodies 1
extrude "Extrude22" add sketch "Sketch11" along normal blind 35 contours L4 L5 L6 L18 bodies 1
sketch "Sketch12" plane through (0, 0, -40) normal (0, 0, -1) x (-1, 0, 0)
  line L0 (-13, 46.5) -> (-13, 5)
  line L1 (-13, 5) -> (-6, 0)
  line L2 (-6, 0) -> (6, 0)
  line L3 (6, 0) -> (13, 5)
  line L4 (13, 5) -> (13, 46.5)
  line L5 (13, 46.5) -> (-13, 46.5)
  line L6 (0, 46.5) -> (0, 41.5) construction
  line L7 (0, 41.5) -> (-42.5, 41.5) construction
  line L8 (-42.5, 41.5) -> (42.5, 41.5) construction
  line L9 (42.5, 41.5) -> (42.5, 17.5) construction
  line L10 (42.5, 17.5) -> (-42.5, 17.5) construction
  line L11 (-42.5, 17.5) -> (-42.5, 41.5) construction
  dimension "d152" = 5
  dimension "d153" = 42.5
  dimension "d154" = 85
  dimension "d155" = 24
  constraint midpoint L5 L6.start
  constraint perpendicular L5 L6
  constraint perpendicular L6 L7
  constraint horizontal L8
  constraint vertical L9
  constraint horizontal L10
  constraint vertical L11
  measures "d152" distance of L6.start L6.end
  measures "d153" distance of L6.end L7.end
  measures "d154" distance of L7.end L8.end
  measures "d155" distance of L7.end L10.end
sketch "Sketch13" plane through (0, 0, -40) normal (0, 0, -1) x (-1, 0, 0)
  line L0 (-13, 46.5) -> (-13, 5)
  line L1 (-13, 5) -> (-6, 0)
  line L2 (-6, 0) -> (6, 0)
  line L3 (6, 0) -> (13, 5)
  line L4 (13, 5) -> (13, 46.5)
  line L5 (13, 46.5) -> (-13, 46.5)
  line L6 (-10.5765, 39.4382) -> (10.4766, 39.4382) construction
  line L7 (10.4766, 39.4382) -> (10.4766, 25.6042) construction
  line L8 (10.4766, 25.6042) -> (-10.6374, 25.6042) construction
  circle A0 centre (10.4766, 39.4382) radius 0.8
  circle A1 centre (-10.5765, 39.4382) radius 0.8
  circle A2 centre (-10.6374, 25.6042) radius 0.8
  circle A3 centre (10.4766, 25.6042) radius 0.8
  dimension "d159" = 1.6
  dimension "d160" = 1.6
  dimension "d161" = 1.6
  dimension "d162" = 1.6
  constraint perpendicular L4 L6
  constraint perpendicular L6 L7
  constraint perpendicular L4 L8
  constraint coincident L6.end L7.start
  constraint coincident L6.start A1.centre
  constraint coincident L8.end A2.centre
  constraint coincident L7.end L8.start
  measures "d159" diameter of A0
  measures "d160" diameter of A1
  measures "d161" diameter of A2
  measures "d162" diameter of A3
extrude "Extrude23" cut sketch "Sketch13" against normal blind 9 contours A0 | A1 | A2 | A3 bodies 1
fillet "Fillet9" radius 3 2 edges at (13, 46.5, -37.5) (-13, 46.5, -37.5) on bodies 1
fillet "Fillet10" radius 3 4 edges at (-13, 5, -32.5) (13, 5, -35.5105) (-6, 0, -32.5) (6, 0, -32.5) on bodies 1
chamfer "Chamfer1" distance 2 distance2 5 1 edges at (0, 16.5, -25) measured on face at (0.0324, 16.5, -26.5679) on bodies 1
fillet "Fillet11" radius 1 1 edges at (0, 16.5, -35) on bodies 1
fillet "Fillet12" radius 5 2 edges at (22.2021, 54, 11.6175) (15.6999, 54, 10.2097) on bodies 4
equation "d92 = ( 29.5 * 2 ) * 1 mm"
equation "d150 = 5 mm + 30 mm"
